Autodesk Inventor part; units mm, degrees
(part 2 of 3)
  line L626 (-3.7114, -1.0079) -> (-3.7114, -1.9201)
  line L627 (-3.7114, -1.9201) -> (-3.9151, -1.9201)
  line L628 (15.624, -5.9598) -> (15.8032, -5.9598)
  line L629 (15.8032, -5.9598) -> (15.0783, -8.4358)
  line L630 (15.0783, -8.4358) -> (14.8991, -8.4358)
  line L631 (14.8991, -8.4358) -> (15.624, -5.9598)
  line L632 (16.8294, -9.4213) -> (17.0005, -9.4213)
  line L633 (17.0005, -9.4213) -> (16.2837, -11.8973)
  line L634 (16.2837, -11.8973) -> (16.1045, -11.8973)
  line L635 (16.1045, -11.8973) -> (16.8294, -9.4213)
  line L636 (16.7006, -8.1166) -> (16.3044, -8.3052) construction
  spline S44 degree 4 poles (16.6258, -6.9128) (16.5928, -6.7161) (16.4312, -6.6396) (16.2892, -6.6526) (16.1527, -6.7477) (16.117, -6.9928) (16.263, -7.1451) (16.5325, -7.2135) (16.7006, -7.2932) (16.8664, -7.4592) (16.9149, -7.8453) (16.7006, -8.1166) (16.3044, -8.3052) (15.9635, -8.063) (15.8692, -7.8103) (15.8602, -7.6295) knots 1 1 1 1 1 2 3 4 5 6 7 8 9 10 11 12 13 13 13 13 13
  line L637 (16.6258, -6.9128) -> (16.5928, -6.7161) construction
  line L638 (16.5928, -6.7161) -> (16.4312, -6.6396) construction
  line L639 (16.4312, -6.6396) -> (16.2892, -6.6526) construction
  line L640 (16.2892, -6.6526) -> (16.1527, -6.7477) construction
  line L641 (16.1527, -6.7477) -> (16.117, -6.9928) construction
  line L642 (16.117, -6.9928) -> (16.263, -7.1451) construction
  line L643 (16.263, -7.1451) -> (16.5325, -7.2135) construction
  line L644 (16.5325, -7.2135) -> (16.7006, -7.2932) construction
  line L645 (16.7006, -7.2932) -> (16.8664, -7.4592) construction
  line L646 (16.8664, -7.4592) -> (16.9149, -7.8453) construction
  line L647 (16.9149, -7.8453) -> (16.7006, -8.1166) construction
  line L648 (16.3044, -8.3052) -> (15.9635, -8.063) construction
  line L649 (15.9635, -8.063) -> (15.8692, -7.8103) construction
  line L650 (15.8692, -7.8103) -> (15.8602, -7.6295) construction
  line L651 (16.3801, -7.4011) -> (16.1104, -7.3258) construction
  spline S45 degree 4 poles (16.072, -7.6295) (16.0903, -7.8128) (16.1895, -7.9615) (16.3888, -8.02) (16.5928, -7.9509) (16.6874, -7.7036) (16.5928, -7.5208) (16.5342, -7.4592) (16.3801, -7.4011) (16.1104, -7.3258) (15.924, -7.1016) (15.9359, -6.9137) (15.9559, -6.7161) (16.0588, -6.563) (16.226, -6.4563) (16.5549, -6.4563) (16.6874, -6.5163) (16.8173, -6.6705) (16.8457, -6.9128) knots 1 1 1 1 1 2 3 4 5 6 7 8 9 10 11 12 13 14 15 16 16 16 16 16
  line L652 (16.072, -7.6295) -> (16.0903, -7.8128) construction
  line L653 (16.0903, -7.8128) -> (16.1895, -7.9615) construction
  line L654 (16.1895, -7.9615) -> (16.3888, -8.02) construction
  line L655 (16.3888, -8.02) -> (16.5928, -7.9509) construction
  line L656 (16.5928, -7.9509) -> (16.6874, -7.7036) construction
  line L657 (16.6874, -7.7036) -> (16.5928, -7.5208) construction
  line L658 (16.5928, -7.5208) -> (16.5342, -7.4592) construction
  line L659 (16.5342, -7.4592) -> (16.3801, -7.4011) construction
  line L660 (16.1104, -7.3258) -> (15.924, -7.1016) construction
  line L661 (15.924, -7.1016) -> (15.9359, -6.9137) construction
  line L662 (15.9359, -6.9137) -> (15.9559, -6.7161) construction
  line L663 (15.9559, -6.7161) -> (16.0588, -6.563) construction
  line L664 (16.0588, -6.563) -> (16.226, -6.4563) construction
  line L665 (16.226, -6.4563) -> (16.5549, -6.4563) construction
  line L666 (16.5549, -6.4563) -> (16.6874, -6.5163) construction
  line L667 (16.6874, -6.5163) -> (16.8173, -6.6705) construction
  line L668 (16.8173, -6.6705) -> (16.8457, -6.9128) construction
  line L669 (16.6258, -6.9128) -> (16.8457, -6.9128)
  line L670 (15.8602, -7.6295) -> (16.072, -7.6295)
  line L671 (12.3499, -9.4213) -> (12.3499, -11.6122)
  line L672 (12.3499, -11.6122) -> (12.5535, -11.6122)
  line L673 (12.5535, -11.6122) -> (12.5535, -10.7624)
  line L674 (13.2295, -11.6122) -> (13.4901, -11.6122)
  line L675 (13.4901, -11.6122) -> (12.7815, -10.7245)
  line L676 (12.7815, -10.7245) -> (13.3598, -9.9507)
  line L677 (13.3598, -9.9507) -> (13.1317, -9.9507)
  line L678 (12.5535, -10.7124) -> (12.5535, -9.4213)
  line L679 (12.5535, -9.4213) -> (12.3499, -9.4213)
  line L680 (12.5535, -10.7124) -> (12.5625, -10.7124)
  line L681 (12.5625, -10.7124) -> (13.1317, -9.9507)
  line L682 (12.5535, -10.7624) -> (12.564, -10.7624)
  line L683 (12.564, -10.7624) -> (13.2295, -11.6122)
  line L684 (19.6312, -4.8847) -> (20.7633, -2.6042)
  line L685 (20.7633, -2.6042) -> (20.5923, -2.6042)
  line L686 (20.5923, -2.6042) -> (19.4602, -4.8847)
  line L687 (19.4602, -4.8847) -> (19.6312, -4.8847)
  circle A1 centre (19.4602, -3.1424) radius 0.3325
  circle A2 centre (19.4602, -3.1424) radius 0.5381
  circle A3 centre (20.7583, -4.3418) radius 0.3325
  circle A4 centre (20.7583, -4.3418) radius 0.5381
  line L688 (10.8197, 1.0564) -> (-20.3114, 1.0564)
  line L689 (-20.3114, 1.0564) -> (-20.3114, 1.2564)
  line L690 (-20.3114, 1.2564) -> (10.8197, 1.2564)
  line L691 (10.8197, 1.2564) -> (10.8197, 1.0564)
  line L692 (-21.284, 2.029) -> (-21.084, 2.029)
  line L693 (-21.084, 2.029) -> (-21.084, 12.0899)
  line L694 (-21.084, 12.0899) -> (-21.284, 12.0899)
  line L695 (-21.284, 12.0899) -> (-21.284, 2.029)
  line L696 (-20.3114, 12.8625) -> (10.8197, 12.8625)
  line L697 (10.8197, 12.8625) -> (10.8197, 13.0625)
  line L698 (10.8197, 13.0625) -> (-20.3114, 13.0625)
  line L699 (-20.3114, 13.0625) -> (-20.3114, 12.8625)
  line L700 (11.5924, 12.0899) -> (11.7924, 12.0899)
  line L701 (11.7924, 12.0899) -> (11.7924, 2.029)
  line L702 (11.7924, 2.029) -> (11.5924, 2.029)
  line L703 (11.5924, 2.029) -> (11.5924, 12.0899)
  line L704 (9.8564, 15.8189) -> (9.8564, 13.8208)
  line L705 (9.9764, 15.8189) -> (9.9764, 13.8208)
  line L706 (10.1798, 16.1424) -> (10.5173, 16.1424)
  line L707 (10.1798, 16.0224) -> (11.4983, 16.0224)
  line L708 (11.1689, 16.1424) -> (11.4983, 16.1424)
  line L709 (11.1689, 16.1424) -> (11.1689, 16.3297)
  line L710 (10.5173, 16.1424) -> (10.5173, 16.3297)
  line L711 (10.5417, 16.3541) -> (11.1444, 16.3541)
  arc A5 (10.1798, 16.1424) -> (9.8564, 15.8189) centre (10.1798, 15.8189) ccw
  arc A6 (10.1798, 16.0224) -> (9.9764, 15.8189) centre (10.1798, 15.8189) ccw
  arc A7 (11.8217, 15.8189) -> (11.4983, 16.1424) centre (11.4983, 15.8189) ccw
  arc A8 (11.7017, 15.8189) -> (11.4983, 16.0224) centre (11.4983, 15.8189) ccw
  arc A9 (9.8564, 13.8208) -> (10.1798, 13.4974) centre (10.1798, 13.8208) ccw
  arc A10 (9.9764, 13.8208) -> (10.1798, 13.6174) centre (10.1798, 13.8208) ccw
  arc A11 (11.4983, 13.6174) -> (11.7017, 13.8208) centre (11.4983, 13.8208) ccw
  arc A12 (11.4983, 13.4974) -> (11.8217, 13.8208) centre (11.4983, 13.8208) ccw
  line L712 (11.7017, 15.8189) -> (11.7017, 13.8208)
  line L713 (11.8217, 15.8189) -> (11.8217, 13.8208)
  line L714 (11.4983, 13.6174) -> (11.039, 13.6174)
  line L715 (11.039, 13.6174) -> (11.039, 13.4974)
  line L716 (11.039, 13.4974) -> (11.4983, 13.4974)
  line L717 (10.1798, 13.6174) -> (10.639, 13.6174)
  line L718 (10.639, 13.6174) -> (10.639, 13.4974)
  line L719 (10.639, 13.4974) -> (10.1798, 13.4974)
  arc A13 (10.5417, 16.3541) -> (10.5173, 16.3297) centre (10.5417, 16.3297) ccw
  arc A14 (11.1689, 16.3297) -> (11.1444, 16.3541) centre (11.1444, 16.3297) ccw
  circle A15 centre (8.2981, 11.6945) radius 0.3325
  circle A16 centre (8.2981, 11.6945) radius 0.5381
  line L720 (9.597, 7.7802) -> (8.7499, 5.345)
  line L721 (8.7499, 5.345) -> (10.4521, 5.345)
  line L722 (10.4521, 5.345) -> (9.597, 7.7802)
  line L723 (8.7499, 4.4979) -> (10.4521, 4.4979)
  line L724 (10.4521, 4.4979) -> (9.597, 2.0627)
  line L725 (9.597, 2.0627) -> (8.7499, 4.4979)
  line L726 (9.3608, 5.295) -> (9.8413, 5.295)
  line L727 (9.8413, 5.295) -> (9.8413, 4.5479)
  line L728 (9.8413, 4.5479) -> (9.3608, 4.5479)
  line L729 (9.3608, 4.5479) -> (9.3608, 5.295)
  line L730 (13.8648, -0.8287) -> (16.3, 0.0184)
  line L731 (16.3, 0.0184) -> (16.3, -1.6839)
  line L732 (16.3, -1.6839) -> (13.8648, -0.8287)
  line L733 (17.8068, 0.0591) -> (20.242, -0.788)
  line L734 (20.242, -0.788) -> (17.8068, -1.6432)
  line L735 (17.8068, -1.6432) -> (17.8068, 0.0591)
  line L736 (16.35, -0.5925) -> (17.7568, -0.5925)
  line L737 (17.7568, -0.5925) -> (17.7568, -1.073)
  line L738 (17.7568, -1.073) -> (16.35, -1.073)
  line L739 (16.35, -1.073) -> (16.35, -0.5925)
  line L740 (-21.0759, -3.4746) -> (-20.8759, -3.4746)
  line L741 (-20.8759, -3.4746) -> (-20.8759, -10.636)
  line L742 (-20.8759, -10.636) -> (-21.0759, -10.636)
  line L743 (-21.0759, -10.636) -> (-21.0759, -3.4746)
  line L744 (-20.1032, -11.2086) -> (-0.5783, -11.2086)
  line L745 (-0.5783, -11.2086) -> (-0.5783, -11.4086)
  line L746 (-0.5783, -11.4086) -> (-20.1032, -11.4086)
  line L747 (-20.1032, -11.4086) -> (-20.1032, -11.2086)
  line L748 (1.167, -11.2086) -> (10.6197, -11.2086)
  line L749 (10.6197, -11.2086) -> (10.6197, -11.4086)
  line L750 (10.6197, -11.4086) -> (1.167, -11.4086)
  line L751 (1.167, -11.4086) -> (1.167, -11.2086)
  line L752 (11.3924, -3.4746) -> (11.5924, -3.4746)
  line L753 (11.5924, -3.4746) -> (11.5924, -10.636)
  line L754 (11.5924, -10.636) -> (11.3924, -10.636)
  line L755 (11.3924, -10.636) -> (11.3924, -3.4746)
  line L756 (1.167, -2.702) -> (10.6197, -2.702)
  line L757 (10.6197, -2.702) -> (10.6197, -2.902)
  line L758 (10.6197, -2.902) -> (1.167, -2.902)
  line L759 (1.167, -2.902) -> (1.167, -2.702)
  line L760 (0.1943, -3.4746) -> (0.3943, -3.4746)
  line L761 (0.3943, -3.4746) -> (0.3943, -10.636)
  line L762 (0.3943, -10.636) -> (0.1943, -10.636)
  line L763 (0.1943, -10.636) -> (0.1943, -3.4746)
  line L764 (-20.1032, -2.702) -> (-0.5783, -2.702)
  line L765 (-0.5783, -2.702) -> (-0.5783, -2.902)
  line L766 (-0.5783, -2.902) -> (-20.1032, -2.902)
  line L767 (-20.1032, -2.902) -> (-20.1032, -2.702)
  line L768 (5.5409, -9.6819) -> (6.2658, -9.6819)
  line L769 (6.2658, -9.6819) -> (6.2658, -10.3987)
  line L770 (6.2658, -10.3987) -> (5.5409, -10.3987)
  line L771 (5.5409, -10.3987) -> (5.5409, -9.6819)
  line L772 (-10.9195, -5.7806) -> (-10.1946, -5.7806)
  line L773 (-10.1946, -5.7806) -> (-10.1946, -6.5055)
  line L774 (-10.1946, -6.5055) -> (-10.9195, -6.5055)
  line L775 (-10.9195, -6.5055) -> (-10.9195, -5.7806)
  line L776 (-10.9195, -7.5236) -> (-10.1946, -7.5236)
  line L777 (-10.1946, -7.5236) -> (-10.1946, -8.2403)
  line L778 (-10.1946, -8.2403) -> (-10.9195, -8.2403)
  line L779 (-10.9195, -8.2403) -> (-10.9195, -7.5236)
  line L780 (-10.9195, -9.6819) -> (-10.1946, -9.6819)
  line L781 (-10.1946, -9.6819) -> (-10.1946, -10.3987)
  line L782 (-10.1946, -10.3987) -> (-10.9195, -10.3987)
  line L783 (-10.9195, -10.3987) -> (-10.9195, -9.6819)
  line L784 (-5.7558, -9.6819) -> (-5.0309, -9.6819)
  line L785 (-5.0309, -9.6819) -> (-5.0309, -10.3987)
  line L786 (-5.0309, -10.3987) -> (-5.7558, -10.3987)
  line L787 (-5.7558, -10.3987) -> (-5.7558, -9.6819)
  line L788 (-19.4714, -3.6467) -> (-17.2723, -3.6467)
  line L789 (-17.2723, -3.6467) -> (-16.9221, -3.997)
  line L790 (-16.9221, -3.997) -> (-17.2397, -4.3146)
  line L791 (-17.2397, -4.3146) -> (-19.4567, -4.3146)
  line L792 (-19.7938, -3.9691) -> (-19.4714, -3.6467)
  line L793 (-19.8786, -4.054) -> (-19.5528, -4.3879)
  line L794 (-19.5528, -4.3879) -> (-19.5528, -6.5964)
  line L795 (-19.5528, -6.5964) -> (-19.9227, -6.9664)
  line L796 (-19.9227, -6.9664) -> (-20.2125, -6.6766)
  line L797 (-20.2125, -6.6766) -> (-20.2125, -4.3879)
  line L798 (-20.2125, -4.3879) -> (-19.8786, -4.054)
  line L799 (-19.8379, -7.0512) -> (-19.504, -6.7173)
  line L800 (-19.504, -6.7173) -> (-17.2397, -6.7173)
  line L801 (-17.2397, -6.7173) -> (-16.9058, -7.0512)
  line L802 (-16.9058, -7.0512) -> (-17.2397, -7.3851)
  line L803 (-17.2397, -7.3851) -> (-19.504, -7.3851)
  line L804 (-19.504, -7.3851) -> (-19.8379, -7.0512)
  line L805 (-19.7938, -3.9691) -> (-19.4567, -4.3146)
  line L806 (-16.8372, -4.0818) -> (-17.199, -4.4436)
  line L807 (-17.199, -4.4436) -> (-17.199, -6.5883)
  line L808 (-17.199, -6.5883) -> (-16.821, -6.9664)
  line L809 (-16.821, -6.9664) -> (-16.5312, -6.6766)
  line L810 (-16.5312, -6.6766) -> (-16.5312, -4.3879)
  line L811 (-16.5312, -4.3879) -> (-16.8372, -4.0818)
  line L812 (-16.821, -7.1361) -> (-17.199, -7.5141)
  line L813 (-17.199, -7.5141) -> (-17.199, -9.7064)
  line L814 (-17.199, -9.7064) -> (-16.8651, -10.0403)
  line L815 (-16.8651, -10.0403) -> (-16.5312, -9.7064)
  line L816 (-16.5312, -9.7064) -> (-16.5312, -7.4259)
  line L817 (-16.5312, -7.4259) -> (-16.821, -7.1361)
  line L818 (-19.9227, -7.1361) -> (-20.2125, -7.4259)
  line L819 (-20.2125, -7.4259) -> (-20.2125, -9.7064)
  line L820 (-20.2125, -9.7064) -> (-19.8786, -10.0403)
  line L821 (-19.8786, -10.0403) -> (-19.5528, -9.7064)
  line L822 (-19.5528, -9.7064) -> (-19.5528, -7.506)
  line L823 (-19.5528, -7.506) -> (-19.9227, -7.1361)
  line L824 (-19.7938, -10.1252) -> (-19.417, -9.739)
  line L825 (-19.417, -9.739) -> (-17.3361, -9.739)
  line L826 (-17.3361, -9.739) -> (-16.9499, -10.1252)
  line L827 (-16.9499, -10.1252) -> (-17.2316, -10.4068)
  line L828 (-17.2316, -10.4068) -> (-19.5121, -10.4068)
  line L829 (-19.5121, -10.4068) -> (-19.7938, -10.1252)
  line L830 (-11.6919, -4.0818) -> (-12.0536, -4.4436)
  line L831 (-11.6756, -7.1361) -> (-12.0536, -7.5141)
  line L832 (-11.7604, -7.0512) -> (-12.0943, -7.3851)
  line L833 (-14.4074, -9.7064) -> (-14.4074, -7.506)
  line L834 (-15.0672, -7.4259) -> (-15.0672, -9.7064)
  line L835 (-14.7774, -7.1361) -> (-15.0672, -7.4259)
  line L836 (-14.4074, -7.506) -> (-14.7774, -7.1361)
  line L837 (-14.3586, -7.3851) -> (-14.6925, -7.0512)
  line L838 (-12.0943, -7.3851) -> (-14.3586, -7.3851)
  line L839 (-11.3858, -6.6766) -> (-11.3858, -4.3879)
  line L840 (-11.6756, -6.9664) -> (-11.3858, -6.6766)
  line L841 (-11.3858, -7.4259) -> (-11.6756, -7.1361)
  line L842 (-11.3858, -9.7064) -> (-11.3858, -7.4259)
  line L843 (-12.0536, -7.5141) -> (-12.0536, -9.7064)
  line L844 (-11.3858, -4.3879) -> (-11.6919, -4.0818)
  line L845 (-14.6484, -3.9691) -> (-14.326, -3.6467)
  line L846 (-14.6484, -3.9691) -> (-14.3113, -4.3146)
  line L847 (-14.7332, -4.054) -> (-14.4074, -4.3879)
  line L848 (-15.0672, -4.3879) -> (-14.7332, -4.054)
  line L849 (-14.326, -3.6467) -> (-12.1269, -3.6467)
  line L850 (-12.1269, -3.6467) -> (-11.7767, -3.997)
  line L851 (-12.0943, -4.3146) -> (-14.3113, -4.3146)
  line L852 (-11.7767, -3.997) -> (-12.0943, -4.3146)
  line L853 (-12.0536, -4.4436) -> (-12.0536, -6.5883)
  line L854 (-14.3586, -6.7173) -> (-12.0943, -6.7173)
  line L855 (-12.0536, -6.5883) -> (-11.6756, -6.9664)
  line L856 (-12.0943, -6.7173) -> (-11.7604, -7.0512)
  line L857 (-14.4074, -4.3879) -> (-14.4074, -6.5964)
  line L858 (-15.0672, -6.6766) -> (-15.0672, -4.3879)
  line L859 (-14.6925, -7.0512) -> (-14.3586, -6.7173)
  line L860 (-14.4074, -6.5964) -> (-14.7774, -6.9664)
  line L861 (-14.7774, -6.9664) -> (-15.0672, -6.6766)
  line L862 (-14.2716, -9.739) -> (-12.1908, -9.739)
  line L863 (-11.7197, -10.0403) -> (-11.3858, -9.7064)
  line L864 (-12.0536, -9.7064) -> (-11.7197, -10.0403)
  line L865 (-12.1908, -9.739) -> (-11.8045, -10.1252)
  line L866 (-12.0862, -10.4068) -> (-14.3667, -10.4068)
  line L867 (-11.8045, -10.1252) -> (-12.0862, -10.4068)
  line L868 (-14.7332, -10.0403) -> (-14.4074, -9.7064)
  line L869 (-14.6484, -10.1252) -> (-14.2716, -9.739)
  line L870 (-15.0672, -9.7064) -> (-14.7332, -10.0403)
  line L871 (-14.3667, -10.4068) -> (-14.6484, -10.1252)
  line L872 (-6.4446, -4.0818) -> (-6.8064, -4.4436)
  line L873 (-6.4284, -7.1361) -> (-6.8064, -7.5141)
  line L874 (-6.5132, -7.0512) -> (-6.8471, -7.3851)
  line L875 (-9.1602, -9.7064) -> (-9.1602, -7.506)
  line L876 (-9.8199, -7.4259) -> (-9.8199, -9.7064)
  line L877 (-9.5301, -7.1361) -> (-9.8199, -7.4259)
  line L878 (-9.1602, -7.506) -> (-9.5301, -7.1361)
  line L879 (-9.1114, -7.3851) -> (-9.4453, -7.0512)
  line L880 (-6.8471, -7.3851) -> (-9.1114, -7.3851)
  line L881 (-6.1386, -6.6766) -> (-6.1386, -4.3879)
  line L882 (-6.4284, -6.9664) -> (-6.1386, -6.6766)
  line L883 (-6.1386, -7.4259) -> (-6.4284, -7.1361)
  line L884 (-6.1386, -9.7064) -> (-6.1386, -7.4259)
  line L885 (-6.8064, -7.5141) -> (-6.8064, -9.7064)
  line L886 (-6.1386, -4.3879) -> (-6.4446, -4.0818)
  line L887 (-9.4012, -3.9691) -> (-9.0788, -3.6467)
  line L888 (-9.4012, -3.9691) -> (-9.0641, -4.3146)
  line L889 (-9.486, -4.054) -> (-9.1602, -4.3879)
  line L890 (-9.8199, -4.3879) -> (-9.486, -4.054)
  line L891 (-9.0788, -3.6467) -> (-6.8797, -3.6467)
  line L892 (-6.8797, -3.6467) -> (-6.5295, -3.997)
  line L893 (-6.8471, -4.3146) -> (-9.0641, -4.3146)
  line L894 (-6.5295, -3.997) -> (-6.8471, -4.3146)
  line L895 (-6.8064, -4.4436) -> (-6.8064, -6.5883)
  line L896 (-9.1114, -6.7173) -> (-6.8471, -6.7173)
  line L897 (-6.8064, -6.5883) -> (-6.4284, -6.9664)
  line L898 (-6.8471, -6.7173) -> (-6.5132, -7.0512)
  line L899 (-9.1602, -4.3879) -> (-9.1602, -6.5964)
  line L900 (-9.8199, -6.6766) -> (-9.8199, -4.3879)
  line L901 (-9.4453, -7.0512) -> (-9.1114, -6.7173)
  line L902 (-9.1602, -6.5964) -> (-9.5301, -6.9664)
  line L903 (-9.5301, -6.9664) -> (-9.8199, -6.6766)
  line L904 (-9.0244, -9.739) -> (-6.9435, -9.739)
  line L905 (-6.4725, -10.0403) -> (-6.1386, -9.7064)
  line L906 (-6.8064, -9.7064) -> (-6.4725, -10.0403)
  line L907 (-6.9435, -9.739) -> (-6.5573, -10.1252)
  line L908 (-6.839, -10.4068) -> (-9.1195, -10.4068)
  line L909 (-6.5573, -10.1252) -> (-6.839, -10.4068)
  line L910 (-9.486, -10.0403) -> (-9.1602, -9.7064)
  line L911 (-9.4012, -10.1252) -> (-9.0244, -9.739)
  line L912 (-9.8199, -9.7064) -> (-9.486, -10.0403)
  line L913 (-9.1195, -10.4068) -> (-9.4012, -10.1252)
  line L914 (-1.2565, -4.0818) -> (-1.6183, -4.4436)
  line L915 (-1.2402, -7.1361) -> (-1.6183, -7.5141)
  line L916 (-1.325, -7.0512) -> (-1.659, -7.3851)
  line L917 (-3.9721, -9.7064) -> (-3.9721, -7.506)
  line L918 (-4.6318, -7.4259) -> (-4.6318, -9.7064)
  line L919 (-4.342, -7.1361) -> (-4.6318, -7.4259)
  line L920 (-3.9721, -7.506) -> (-4.342, -7.1361)
  line L921 (-3.9232, -7.3851) -> (-4.2571, -7.0512)
  line L922 (-1.659, -7.3851) -> (-3.9232, -7.3851)
  line L923 (-0.9504, -6.6766) -> (-0.9504, -4.3879)
  line L924 (-1.2402, -6.9664) -> (-0.9504, -6.6766)
  line L925 (-0.9504, -7.4259) -> (-1.2402, -7.1361)
  line L926 (-0.9504, -9.7064) -> (-0.9504, -7.4259)
  line L927 (-1.6183, -7.5141) -> (-1.6183, -9.7064)
  line L928 (-0.9504, -4.3879) -> (-1.2565, -4.0818)
  line L929 (-4.213, -3.9691) -> (-3.8906, -3.6467)
  line L930 (-4.213, -3.9691) -> (-3.8759, -4.3146)
  line L931 (-4.2979, -4.054) -> (-3.9721, -4.3879)
  line L932 (-4.6318, -4.3879) -> (-4.2979, -4.054)
  line L933 (-3.8906, -3.6467) -> (-1.6916, -3.6467)
  line L934 (-1.6916, -3.6467) -> (-1.3413, -3.997)
  line L935 (-1.659, -4.3146) -> (-3.8759, -4.3146)
  line L936 (-1.3413, -3.997) -> (-1.659, -4.3146)
  line L937 (-1.6183, -4.4436) -> (-1.6183, -6.5883)
  line L938 (-3.9232, -6.7173) -> (-1.659, -6.7173)
  line L939 (-1.6183, -6.5883) -> (-1.2402, -6.9664)
  line L940 (-1.659, -6.7173) -> (-1.325, -7.0512)
  line L941 (-3.9721, -4.3879) -> (-3.9721, -6.5964)
  line L942 (-4.6318, -6.6766) -> (-4.6318, -4.3879)
  line L943 (-4.2571, -7.0512) -> (-3.9232, -6.7173)
  line L944 (-3.9721, -6.5964) -> (-4.342, -6.9664)
  line L945 (-4.342, -6.9664) -> (-4.6318, -6.6766)
  line L946 (-3.8362, -9.739) -> (-1.7554, -9.739)
  line L947 (-1.2843, -10.0403) -> (-0.9504, -9.7064)
  line L948 (-1.6183, -9.7064) -> (-1.2843, -10.0403)
  line L949 (-1.7554, -9.739) -> (-1.3692, -10.1252)
  line L950 (-1.6508, -10.4068) -> (-3.9313, -10.4068)
  line L951 (-1.3692, -10.1252) -> (-1.6508, -10.4068)
  line L952 (-4.2979, -10.0403) -> (-3.9721, -9.7064)
  line L953 (-4.213, -10.1252) -> (-3.8362, -9.739)
  line L954 (-4.6318, -9.7064) -> (-4.2979, -10.0403)
  line L955 (-3.9313, -10.4068) -> (-4.213, -10.1252)
  line L956 (4.8439, -4.0818) -> (4.4821, -4.4436)
  line L957 (4.8602, -7.1361) -> (4.4821, -7.5141)
  line L958 (4.7753, -7.0512) -> (4.4414, -7.3851)
  line L959 (2.1283, -9.7064) -> (2.1283, -7.506)
  line L960 (1.4686, -7.4259) -> (1.4686, -9.7064)
  line L961 (1.7584, -7.1361) -> (1.4686, -7.4259)
  line L962 (2.1283, -7.506) -> (1.7584, -7.1361)
  line L963 (2.1772, -7.3851) -> (1.8432, -7.0512)
  line L964 (4.4414, -7.3851) -> (2.1772, -7.3851)
  line L965 (5.15, -6.6766) -> (5.15, -4.3879)
  line L966 (4.8602, -6.9664) -> (5.15, -6.6766)
  line L967 (5.15, -7.4259) -> (4.8602, -7.1361)
  line L968 (5.15, -9.7064) -> (5.15, -7.4259)
  line L969 (4.4821, -7.5141) -> (4.4821, -9.7064)
  line L970 (5.15, -4.3879) -> (4.8439, -4.0818)
  line L971 (1.8874, -3.9691) -> (2.2097, -3.6467)
  line L972 (1.8874, -3.9691) -> (2.2244, -4.3146)
  line L973 (1.8025, -4.054) -> (2.1283, -4.3879)
  line L974 (1.4686, -4.3879) -> (1.8025, -4.054)
  line L975 (2.2097, -3.6467) -> (4.4088, -3.6467)
  line L976 (4.4088, -3.6467) -> (4.759, -3.997)
  line L977 (4.4414, -4.3146) -> (2.2244, -4.3146)
  line L978 (4.759, -3.997) -> (4.4414, -4.3146)
  line L979 (4.4821, -4.4436) -> (4.4821, -6.5883)
  line L980 (2.1772, -6.7173) -> (4.4414, -6.7173)
  line L981 (4.4821, -6.5883) -> (4.8602, -6.9664)
  line L982 (4.4414, -6.7173) -> (4.7753, -7.0512)
  line L983 (2.1283, -4.3879) -> (2.1283, -6.5964)
  line L984 (1.4686, -6.6766) -> (1.4686, -4.3879)
  line L985 (1.8432, -7.0512) -> (2.1772, -6.7173)
  line L986 (2.1283, -6.5964) -> (1.7584, -6.9664)
  line L987 (1.7584, -6.9664) -> (1.4686, -6.6766)
  line L988 (2.2642, -9.739) -> (4.345, -9.739)
  line L989 (4.816, -10.0403) -> (5.15, -9.7064)
  line L990 (4.4821, -9.7064) -> (4.816, -10.0403)
  line L991 (4.345, -9.739) -> (4.7312, -10.1252)
  line L992 (4.4495, -10.4068) -> (2.169, -10.4068)
  line L993 (4.7312, -10.1252) -> (4.4495, -10.4068)
  line L994 (1.8025, -10.0403) -> (2.1283, -9.7064)
  line L995 (1.8874, -10.1252) -> (2.2642, -9.739)
  line L996 (1.4686, -9.7064) -> (1.8025, -10.0403)
  line L997 (2.169, -10.4068) -> (1.8874, -10.1252)
  line L998 (10.032, -4.0818) -> (9.6703, -4.4436)
  line L999 (10.0483, -7.1361) -> (9.6703, -7.5141)
  line L1000 (9.9635, -7.0512) -> (9.6295, -7.3851)
  line L1001 (7.3164, -9.7064) -> (7.3164, -7.506)
  line L1002 (6.6567, -7.4259) -> (6.6567, -9.7064)
  line L1003 (6.9465, -7.1361) -> (6.6567, -7.4259)
  line L1004 (7.3164, -7.506) -> (6.9465, -7.1361)
  line L1005 (7.3653, -7.3851) -> (7.0314, -7.0512)
  line L1006 (9.6295, -7.3851) -> (7.3653, -7.3851)
  line L1007 (10.3381, -6.6766) -> (10.3381, -4.3879)
  line L1008 (10.0483, -6.9664) -> (10.3381, -6.6766)
  line L1009 (10.3381, -7.4259) -> (10.0483, -7.1361)
  line L1010 (10.3381, -9.7064) -> (10.3381, -7.4259)
  line L1011 (9.6703, -7.5141) -> (9.6703, -9.7064)
  line L1012 (10.3381, -4.3879) -> (10.032, -4.0818)
  line L1013 (7.0755, -3.9691) -> (7.3979, -3.6467)
  line L1014 (7.0755, -3.9691) -> (7.4126, -4.3146)
  line L1015 (6.9907, -4.054) -> (7.3164, -4.3879)
  line L1016 (6.6567, -4.3879) -> (6.9907, -4.054)
  line L1017 (7.3979, -3.6467) -> (9.597, -3.6467)
  line L1018 (9.597, -3.6467) -> (9.9472, -3.997)
  line L1019 (9.6295, -4.3146) -> (7.4126, -4.3146)
  line L1020 (9.9472, -3.997) -> (9.6295, -4.3146)
  line L1021 (9.6703, -4.4436) -> (9.6703, -6.5883)
  line L1022 (7.3653, -6.7173) -> (9.6295, -6.7173)
  line L1023 (9.6703, -6.5883) -> (10.0483, -6.9664)
  line L1024 (9.6295, -6.7173) -> (9.9635, -7.0512)
  line L1025 (7.3164, -4.3879) -> (7.3164, -6.5964)
  line L1026 (6.6567, -6.6766) -> (6.6567, -4.3879)
  line L1027 (7.0314, -7.0512) -> (7.3653, -6.7173)
  line L1028 (7.3164, -6.5964) -> (6.9465, -6.9664)
  line L1029 (6.9465, -6.9664) -> (6.6567, -6.6766)
  line L1030 (7.4523, -9.739) -> (9.5331, -9.739)
  line L1031 (10.0042, -10.0403) -> (10.3381, -9.7064)
  line L1032 (9.6703, -9.7064) -> (10.0042, -10.0403)
  line L1033 (9.5331, -9.739) -> (9.9193, -10.1252)
  line L1034 (9.6377, -10.4068) -> (7.3572, -10.4068)
  line L1035 (9.9193, -10.1252) -> (9.6377, -10.4068)
  line L1036 (6.9907, -10.0403) -> (7.3164, -9.7064)
  line L1037 (7.0755, -10.1252) -> (7.4523, -9.739)
  line L1038 (6.6567, -9.7064) -> (6.9907, -10.0403)
  line L1039 (7.3572, -10.4068) -> (7.0755, -10.1252)
  line L1040 (8.8351, 11.1064) -> (8.8351, 8.9128)
  line L1041 (9.3135, 11.0282) -> (9.3135, 8.9574)
  line L1042 (9.3986, 11.5912) -> (10.3586, 11.5912)
  line L1043 (9.4283, 11.1129) -> (10.3586, 11.1129)
  line L1044 (8.8351, 11.1064) -> (8.9706, 11.5358) construction
  line L1045 (8.9706, 11.5358) -> (9.3986, 11.5912) construction
  spline S46 degree 2 poles (8.8351, 11.1064) (8.9706, 11.5358) (9.3986, 11.5912) knots 1 1 1 2 2 2
  line L1046 (9.3135, 11.0282) -> (9.3594, 11.1062) construction
  line L1047 (9.3594, 11.1062) -> (9.4283, 11.1129) construction
  spline S47 degree 2 poles (9.3135, 11.0282) (9.3594, 11.1062) (9.4283, 11.1129) knots 1 1 1 2 2 2
  line L1048 (8.8351, 8.9128) -> (8.9277, 8.4536) construction
  line L1049 (8.9277, 8.4536) -> (9.3729, 8.3522) construction
  spline S48 degree 2 poles (8.8351, 8.9128) (8.9277, 8.4536) (9.3729, 8.3522) knots 1 1 1 2 2 2
  line L1050 (9.3135, 8.9574) -> (9.3317, 8.865) construction
  line L1051 (9.3317, 8.865) -> (9.4306, 8.8306) construction
  spline S49 degree 2 poles (9.3135, 8.9574) (9.3317, 8.865) (9.4306, 8.8306) knots 1 1 1 2 2 2
  line L1052 (10.386, 8.8306) -> (10.5862, 8.7305) construction
  line L1053 (10.5862, 8.7305) -> (10.5862, 8.4536) construction
  line L1054 (10.5862, 8.4536) -> (10.386, 8.3522) construction
  spline S50 degree 3 poles (10.386, 8.8306) (10.5862, 8.7305) (10.5862, 8.4536) (10.386, 8.3522) knots 1 1 1 1 2 2 2 2
  line L1055 (10.3586, 11.5912) -> (10.611, 11.5234) construction
  line L1056 (10.611, 11.5234) -> (10.611, 11.1907) construction
  line L1057 (10.611, 11.1907) -> (10.3586, 11.1129) construction
  spline S51 degree 3 poles (10.3586, 11.5912) (10.611, 11.5234) (10.611, 11.1907) (10.3586, 11.1129) knots 1 1 1 1 2 2 2 2
  line L1058 (9.4306, 8.8306) -> (10.386, 8.8306)
  line L1059 (10.386, 8.3522) -> (9.3729, 8.3522)
  line L1060 (10.1264, 15.1719) -> (11.511, 15.8398)
  line L1061 (10.1264, 15.7828) -> (10.1264, 15.1719)
  line L1062 (11.4214, 15.8724) -> (10.2567, 15.8724)
  line L1063 (10.1264, 14.8158) -> (11.5517, 15.5)
  line L1064 (11.5517, 15.5) -> (11.5517, 14.824)
  line L1065 (11.5517, 14.824) -> (10.1264, 14.1398)
  line L1066 (10.1264, 14.1398) -> (10.1264, 14.8158)
  line L1067 (10.1671, 13.8) -> (11.5517, 14.4679)
  line L1068 (10.2567, 13.7674) -> (11.4214, 13.7674)
  line L1069 (10.1264, 15.7828) -> (10.1419, 15.8725) construction
  line L1070 (10.1419, 15.8725) -> (10.2567, 15.8724) construction
  spline S52 degree 2 poles (10.1264, 15.7828) (10.1419, 15.8725) (10.2567, 15.8724) knots 1 1 1 2 2 2
  line L1071 (11.4214, 15.8724) -> (11.4945, 15.8725) construction
  line L1072 (11.4945, 15.8725) -> (11.511, 15.8398) construction
  spline S53 degree 2 poles (11.4214, 15.8724) (11.4945, 15.8725) (11.511, 15.8398) knots 1 1 1 2 2 2
  line L1073 (11.5517, 14.4679) -> (11.5517, 13.8733)
  line L1074 (11.5517, 13.8733) -> (11.5412, 13.7747) construction
  line L1075 (11.5412, 13.7747) -> (11.4214, 13.7674) construction
  spline S54 degree 2 poles (11.5517, 13.8733) (11.5412, 13.7747) (11.4214, 13.7674) knots 1 1 1 2 2 2
  line L1076 (10.1671, 13.8) -> (10.2004, 13.7674) construction
  line L1077 (10.2004, 13.7674) -> (10.2567, 13.7674) construction
  spline S55 degree 2 poles (10.1671, 13.8) (10.2004, 13.7674) (10.2567, 13.7674) knots 1 1 1 2 2 2
  circle A17 centre (14.8258, 15.2163) radius 0.3393
  arc A18 (13.882, 16.4787) -> (13.482, 16.0787) centre (13.882, 16.0787) ccw
  arc A19 (16.1697, 16.0787) -> (15.7697, 16.4787) centre (15.7697, 16.0787) ccw
  arc A20 (15.7697, 13.9539) -> (16.1697, 14.3539) centre (15.7697, 14.3539) ccw
  arc A21 (13.482, 14.3539) -> (13.882, 13.9539) centre (13.882, 14.3539) ccw
  line L1078 (13.882, 16.4787) -> (15.7697, 16.4787)
  line L1079 (16.1697, 16.0787) -> (16.1697, 14.3539)
  line L1080 (15.7697, 13.9539) -> (13.882, 13.9539)
  line L1081 (13.482, 16.0787) -> (13.482, 14.3539)
  arc A22 (18.3199, 14.3132) -> (18.7199, 13.9132) centre (18.7199, 14.3132) ccw
  line L1082 (18.3199, 16.038) -> (18.3199, 14.3132)
  arc A23 (18.7199, 16.438) -> (18.3199, 16.038) centre (18.7199, 16.038) ccw
  line L1083 (20.6076, 13.9132) -> (18.7199, 13.9132)
  line L1084 (18.7199, 16.438) -> (20.6076, 16.438)
  arc A24 (20.6076, 13.9132) -> (21.0076, 14.3132) centre (20.6076, 14.3132) ccw
  line L1085 (21.0076, 16.038) -> (21.0076, 14.3132)
  arc A25 (21.0076, 16.038) -> (20.6076, 16.438) centre (20.6076, 16.038) ccw
  line L1086 (19.4351, 14.4795) -> (19.8604, 14.4795)
  line L1087 (19.8604, 14.4795) -> (19.8604, 14.113)
  line L1088 (19.8604, 14.113) -> (19.4351, 14.113)
  line L1089 (19.4351, 14.113) -> (19.4351, 14.4795)
  line L1090 (19.4125, 15.6158) -> (19.4125, 16.0107)
  line L1091 (19.4125, 16.0107) -> (19.8849, 16.0107)
  line L1092 (19.8849, 16.0107) -> (19.8849, 15.5096)
  line L1093 (19.8849, 15.5096) -> (19.7772, 14.6017)
  line L1094 (19.7772, 14.6017) -> (19.5328, 14.6017)
  line L1095 (19.5328, 14.6017) -> (19.4125, 15.6158)
  line L1096 (5.0034, 14.1331) -> (5.6549, 14.5403)
  line L1097 (5.6549, 14.5403) -> (5.6549, 13.848)
  line L1098 (5.6549, 13.848) -> (5.0034, 13.848)
  line L1099 (5.0034, 13.848) -> (5.0034, 14.1331)
  line L1100 (5.997, 14.7602) -> (6.6486, 15.1756)
  line L1101 (6.6486, 15.1756) -> (6.6486, 13.848)
  line L1102 (6.6486, 13.848) -> (5.997, 13.848)
  line L1103 (5.997, 13.848) -> (5.997, 14.7602)
  line L1104 (6.9907, 15.3874) -> (7.6422, 15.8027)
  line L1105 (7.6422, 15.8027) -> (7.6422, 13.848)
  line L1106 (7.6422, 13.848) -> (6.9907, 13.848)
  line L1107 (6.9907, 13.848) -> (6.9907, 15.3874)
  line L1108 (7.9843, 16.0226) -> (8.6359, 16.4266)
  line L1109 (8.6359, 16.4266) -> (8.6359, 13.848)
  line L1110 (8.6359, 13.848) -> (7.9843, 13.848)
  line L1111 (7.9843, 13.848) -> (7.9843, 16.0226)
  line L1112 (14.774, 4.2212) -> (14.774, 4.6384)
  line L1113 (14.774, 4.6384) -> (14.4512, 5.0436)
  line L1114 (14.4512, 5.0436) -> (14.545, 5.1184)
  line L1115 (14.545, 5.1184) -> (14.774, 4.831)
  line L1116 (14.774, 4.831) -> (14.774, 5.2309)
  line L1117 (14.774, 5.2309) -> (14.894, 5.2309)
  line L1118 (14.894, 5.2309) -> (14.894, 4.8352)
  line L1119 (14.894, 4.8352) -> (15.114, 5.1174)
  line L1120 (15.114, 5.1174) -> (15.2086, 5.0436)
  line L1121 (15.2086, 5.0436) -> (14.894, 4.64)
  line L1122 (14.894, 4.64) -> (14.894, 4.2212)
  circle A26 centre (14.834, 3.9115) radius 0.1964
  line L1123 (13.9297, 4.757) -> (14.0409, 4.802)
  line L1124 (14.2331, 4.3277) -> (14.5958, 4.1183)
  line L1125 (14.0409, 4.802) -> (14.2331, 4.3277)
  line L1126 (14.064, 4.4253) -> (13.9297, 4.757)
  line L1127 (13.7213, 4.6232) -> (14.064, 4.4253)
  line L1128 (13.6613, 4.5193) -> (13.7213, 4.6232)
  line L1129 (14.0077, 4.3193) -> (13.6613, 4.5193)
  line L1130 (13.6443, 4.2647) -> (14.0077, 4.3193)
  line L1131 (14.5358, 4.0144) -> (14.1745, 4.223)
  line L1132 (14.1745, 4.223) -> (13.6621, 4.1461)
  line L1133 (13.6621, 4.1461) -> (13.6443, 4.2647)
  line L1134 (13.6496, 3.5511) -> (13.6662, 3.6699)
  line L1135 (14.1731, 3.5992) -> (14.5358, 3.8086)
  line L1136 (13.6662, 3.6699) -> (14.1731, 3.5992)
  line L1137 (14.004, 3.5016) -> (13.6496, 3.5511)
  line L1138 (13.6613, 3.3038) -> (14.004, 3.5016)
  line L1139 (13.7213, 3.1998) -> (13.6613, 3.3038)
  line L1140 (14.0677, 3.3998) -> (13.7213, 3.1998)
  line L1141 (13.9333, 3.0578) -> (14.0677, 3.3998)
  line L1142 (14.5958, 3.7047) -> (14.2345, 3.4961)
  line L1143 (14.2345, 3.4961) -> (14.0449, 3.0139)
  line L1144 (14.0449, 3.0139) -> (13.9333, 3.0578)
  line L1145 (14.554, 2.7056) -> (14.4593, 2.7794)
  line L1146 (14.774, 3.183) -> (14.774, 3.6018)
  line L1147 (14.4593, 2.7794) -> (14.774, 3.183)
  line L1148 (14.774, 2.9878) -> (14.554, 2.7056)
  line L1149 (14.774, 2.5921) -> (14.774, 2.9878)
  line L1150 (14.894, 2.5921) -> (14.774, 2.5921)
  line L1151 (14.894, 2.992) -> (14.894, 2.5921)
  line L1152 (15.1229, 2.7046) -> (14.894, 2.992)
  line L1153 (14.894, 3.6018) -> (14.894, 3.1846)
  line L1154 (14.894, 3.1846) -> (15.2168, 2.7794)
  line L1155 (15.2168, 2.7794) -> (15.1229, 2.7046)
  line L1156 (15.7383, 3.0661) -> (15.6271, 3.021)
  line L1157 (15.4349, 3.4953) -> (15.0722, 3.7047)
  line L1158 (15.6271, 3.021) -> (15.4349, 3.4953)
  line L1159 (15.6039, 3.3977) -> (15.7383, 3.0661)
  line L1160 (15.9466, 3.1998) -> (15.6039, 3.3977)
  line L1161 (16.0066, 3.3038) -> (15.9466, 3.1998)
  line L1162 (15.6603, 3.5037) -> (16.0066, 3.3038)
  line L1163 (16.0236, 3.5583) -> (15.6603, 3.5037)
  line L1164 (15.1322, 3.8086) -> (15.4935, 3.6)
  line L1165 (15.4935, 3.6) -> (16.0058, 3.677)
  line L1166 (16.0058, 3.677) -> (16.0236, 3.5583)
  line L1167 (16.0183, 4.272) -> (16.0017, 4.1531)
  line L1168 (15.4949, 4.2238) -> (15.1322, 4.0144)
  line L1169 (16.0017, 4.1531) -> (15.4949, 4.2238)
  line L1170 (15.6639, 4.3214) -> (16.0183, 4.272)
  line L1171 (16.0066, 4.5193) -> (15.6639, 4.3214)
  line L1172 (15.9466, 4.6232) -> (16.0066, 4.5193)
  line L1173 (15.6003, 4.4232) -> (15.9466, 4.6232)
  line L1174 (15.7347, 4.7652) -> (15.6003, 4.4232)
  line L1175 (15.0722, 4.1183) -> (15.4335, 4.3269)
  line L1176 (15.4335, 4.3269) -> (15.623, 4.8091)
  line L1177 (15.623, 4.8091) -> (15.7347, 4.7652)
  arc A27 (13.9257, 16.0823) -> (13.9127, 14.3642) centre (14.8258, 15.2163) ccw
  arc A28 (14.0531, 15.9338) -> (14.0463, 14.5062) centre (14.8258, 15.2163) ccw
  arc A29 (14.2345, 15.8133) -> (14.221, 14.633) centre (14.8258, 15.2163) ccw
  arc A30 (14.3831, 15.6892) -> (14.327, 14.803) centre (14.8258, 15.2163) ccw
  line L1178 (14.0463, 14.5062) -> (14.1218, 14.4228) construction
  line L1179 (14.1218, 14.4228) -> (14.1126, 14.3627) construction
  line L1180 (14.1126, 14.3627) -> (14.0656, 14.3065) construction
  line L1181 (14.0656, 14.3065) -> (14.0039, 14.3026) construction
  line L1182 (14.0039, 14.3026) -> (13.9661, 14.3098) construction
  line L1183 (13.9661, 14.3098) -> (13.9127, 14.3642) construction
  spline S56 degree 4 poles (14.0463, 14.5062) (14.1218, 14.4228) (14.1126, 14.3627) (14.0656, 14.3065) (14.0039, 14.3026) (13.9661, 14.3098) (13.9127, 14.3642) knots 1 1 1 1 1 2 3 4 4 4 4 4
  line L1184 (14.221, 14.633) -> (14.287, 14.5715) construction
  line L1185 (14.287, 14.5715) -> (14.3743, 14.6118) construction
  line L1186 (14.3743, 14.6118) -> (14.4113, 14.6542) construction
  line L1187 (14.4113, 14.6542) -> (14.4121, 14.7281) construction
  line L1188 (14.4121, 14.7281) -> (14.327, 14.803) construction
  spline S57 degree 4 poles (14.221, 14.633) (14.287, 14.5715) (14.3743, 14.6118) (14.4113, 14.6542) (14.4121, 14.7281) (14.327, 14.803) knots 1 1 1 1 1 2 3 3 3 3 3
  line L1189 (14.2345, 15.8133) -> (14.3224, 15.8802) construction
  line L1190 (14.3224, 15.8802) -> (14.4174, 15.7895) construction
  line L1191 (14.4174, 15.7895) -> (14.4151, 15.7335) construction
  line L1192 (14.4151, 15.7335) -> (14.3831, 15.6892) construction
  spline S58 degree 4 poles (14.2345, 15.8133) (14.3224, 15.8802) (14.4174, 15.7895) (14.4151, 15.7335) (14.3831, 15.6892) knots 1 1 1 1 1 2 2 2 2 2
  line L1193 (13.9257, 16.0823) -> (14.0005, 16.1538) construction
  line L1194 (14.0005, 16.1538) -> (14.0891, 16.1176) construction
  line L1195 (14.0891, 16.1176) -> (14.1126, 16.0648) construction
  line L1196 (14.1126, 16.0648) -> (14.1218, 16.0014) construction
  line L1197 (14.1218, 16.0014) -> (14.0531, 15.9338) construction
  spline S59 degree 4 poles (13.9257, 16.0823) (14.0005, 16.1538) (14.0891, 16.1176) (14.1126, 16.0648) (14.1218, 16.0014) (14.0531, 15.9338) knots 1 1 1 1 1 2 3 3 3 3 3
  line L1198 (15.5391, 16.0699) -> (15.5861, 16.1262) construction
  spline S60 degree 4 poles (15.6054, 15.9264) (15.5298, 16.0098) (15.5391, 16.0699) (15.5861, 16.1262) (15.6478, 16.13) (15.6856, 16.1228) (15.739, 16.0685) knots 1 1 1 1 1 2 3 4 4 4 4 4
  line L1199 (15.6054, 15.9264) -> (15.5298, 16.0098) construction
  line L1200 (15.5298, 16.0098) -> (15.5391, 16.0699) construction
  line L1201 (15.5861, 16.1262) -> (15.6478, 16.13) construction
  line L1202 (15.6478, 16.13) -> (15.6856, 16.1228) construction
  line L1203 (15.6856, 16.1228) -> (15.739, 16.0685) construction
  line L1204 (15.4306, 15.7997) -> (15.3646, 15.8611) construction
  spline S61 degree 4 poles (15.4306, 15.7997) (15.3646, 15.8611) (15.2774, 15.8209) (15.2404, 15.7785) (15.2396, 15.7045) (15.3246, 15.6296) knots 1 1 1 1 1 2 3 3 3 3 3
  line L1205 (15.3646, 15.8611) -> (15.2774, 15.8209) construction
  line L1206 (15.2774, 15.8209) -> (15.2404, 15.7785) construction
  line L1207 (15.2404, 15.7785) -> (15.2396, 15.7045) construction
  line L1208 (15.2396, 15.7045) -> (15.3246, 15.6296) construction
  line L1209 (15.4172, 14.6193) -> (15.3292, 14.5524) construction
  spline S62 degree 4 poles (15.4172, 14.6193) (15.3292, 14.5524) (15.2343, 14.6431) (15.2366, 14.6991) (15.2686, 14.7434) knots 1 1 1 1 1 2 2 2 2 2
  line L1210 (15.3292, 14.5524) -> (15.2343, 14.6431) construction
  line L1211 (15.2343, 14.6431) -> (15.2366, 14.6991) construction
  line L1212 (15.2366, 14.6991) -> (15.2686, 14.7434) construction
  arc A31 (15.7259, 14.3504) -> (15.739, 16.0685) centre (14.8258, 15.2163) ccw
  arc A32 (15.5986, 14.4988) -> (15.6054, 15.9264) centre (14.8258, 15.2163) ccw
  arc A33 (15.4172, 14.6193) -> (15.4306, 15.7997) centre (14.8258, 15.2163) ccw
  arc A34 (15.2686, 14.7434) -> (15.3246, 15.6296) centre (14.8258, 15.2163) ccw
  line L1213 (15.7259, 14.3504) -> (15.6512, 14.2789) construction
  spline S63 degree 4 poles (15.7259, 14.3504) (15.6512, 14.2789) (15.5626, 14.3151) (15.5391, 14.3678) (15.5298, 14.4313) (15.5986, 14.4988) knots 1 1 1 1 1 2 3 3 3 3 3
  line L1214 (15.6512, 14.2789) -> (15.5626, 14.3151) construction
  line L1215 (15.5626, 14.3151) -> (15.5391, 14.3678) construction
  line L1216 (15.5391, 14.3678) -> (15.5298, 14.4313) construction
  line L1217 (15.5298, 14.4313) -> (15.5986, 14.4988) construction
  line L1218 (14.7118, -10.7245) -> (14.7118, -11.6041)
  line L1219 (14.8991, -11.6041) -> (14.7118, -11.6041)
  line L1220 (14.8991, -10.7978) -> (14.8991, -11.6041)
  line L1221 (15.8195, -10.7245) -> (15.8195, -11.6041)
  line L1222 (16.0164, -11.6041) -> (16.0164, -10.7345)
  line L1223 (15.8195, -11.6041) -> (16.0164, -11.6041)
  line L1224 (13.5716, -11.6041) -> (13.5716, -9.9507)
  line L1225 (13.7752, -10.2873) -> (13.7752, -10.6919) construction
  spline S64 degree 4 poles (14.7118, -10.7245) (14.7118, -10.2526) (14.3999, -10.0436) (14.0728, -10.0436) (13.7752, -10.2873) (13.7752, -10.6919) knots 1 1 1 1 1 2 3 3 3 3 3
  line L1226 (14.7118, -10.7245) -> (14.7118, -10.2526) construction
  line L1227 (14.7118, -10.2526) -> (14.3999, -10.0436) construction
  line L1228 (14.3999, -10.0436) -> (14.0728, -10.0436) construction
  line L1229 (14.0728, -10.0436) -> (13.7752, -10.2873) construction
  line L1230 (13.7752, -10.6919) -> (13.7752, -11.6041)
  line L1231 (13.7752, -11.6041) -> (13.5716, -11.6041)
  line L1232 (13.5716, -9.9507) -> (13.7752, -9.9507)
  line L1233 (13.7752, -9.9507) -> (13.7752, -10.138)
  line L1234 (14.0728, -9.8243) -> (14.584, -9.8402) construction
  spline S65 degree 3 poles (13.7752, -10.138) (14.0728, -9.8243) (14.584, -9.8402) (14.834, -10.2113) knots 1 1 1 1 2 2 2 2
  line L1235 (13.7752, -10.138) -> (14.0728, -9.8243) construction
  line L1236 (14.584, -9.8402) -> (14.834, -10.2113) construction
  line L1237 (16.0164, -10.1018) -> (16.0164, -10.7345) construction
  spline S66 degree 4 poles (14.834, -10.2113) (15.1227, -9.7823) (15.8128, -9.7823) (16.0164, -10.1018) (16.0164, -10.7345) knots 1 1 1 1 1 2 2 2 2 2
  line L1238 (14.834, -10.2113) -> (15.1227, -9.7823) construction
  line L1239 (15.1227, -9.7823) -> (15.8128, -9.7823) construction
  line L1240 (15.8128, -9.7823) -> (16.0164, -10.1018) construction
  line L1241 (15.8195, -10.7245) -> (15.8195, -10.2738) construction
  spline S67 degree 4 poles (15.8195, -10.7245) (15.8195, -10.2738) (15.5309, -10.0648) (15.2037, -10.0648) (14.8991, -10.2738) (14.8991, -10.7978) knots 1 1 1 1 1 2 3 3 3 3 3
  line L1242 (15.8195, -10.2738) -> (15.5309, -10.0648) construction
  line L1243 (15.5309, -10.0648) -> (15.2037, -10.0648) construction
  line L1244 (15.2037, -10.0648) -> (14.8991, -10.2738) construction
  line L1245 (14.8991, -10.2738) -> (14.8991, -10.7978) construction
  line L1246 (13.5062, -7.2717) -> (13.5062, -8.1513)
  line L1247 (13.6935, -8.1513) -> (13.5062, -8.1513)
  line L1248 (13.6935, -7.345) -> (13.6935, -8.1513)
  line L1249 (14.6139, -7.2717) -> (14.6139, -8.1513)
  line L1250 (14.8107, -8.1513) -> (14.8107, -7.2817)
  line L1251 (14.6139, -8.1513) -> (14.8107, -8.1513)
  line L1252 (12.3659, -8.1513) -> (12.3659, -6.4979)
  line L1253 (12.5695, -6.8345) -> (12.5695, -7.2391) construction
  spline S68 degree 4 poles (13.5062, -7.2717) (13.5062, -6.7998) (13.1943, -6.5908) (12.8671, -6.5908) (12.5695, -6.8345) (12.5695, -7.2391) knots 1 1 1 1 1 2 3 3 3 3 3
  line L1254 (13.5062, -7.2717) -> (13.5062, -6.7998) construction
  line L1255 (13.5062, -6.7998) -> (13.1943, -6.5908) construction
  line L1256 (13.1943, -6.5908) -> (12.8671, -6.5908) construction
  line L1257 (12.8671, -6.5908) -> (12.5695, -6.8345) construction
  line L1258 (12.5695, -7.2391) -> (12.5695, -8.1513)
  line L1259 (12.5695, -8.1513) -> (12.3659, -8.1513)
  line L1260 (12.3659, -6.4979) -> (12.5695, -6.4979)
  line L1261 (12.5695, -6.4979) -> (12.5695, -6.6852)
  line L1262 (12.8671, -6.3715) -> (13.3783, -6.3874) construction
  spline S69 degree 3 poles (12.5695, -6.6852) (12.8671, -6.3715) (13.3783, -6.3874) (13.6283, -6.7585) knots 1 1 1 1 2 2 2 2
  line L1263 (12.5695, -6.6852) -> (12.8671, -6.3715) construction
  line L1264 (13.3783, -6.3874) -> (13.6283, -6.7585) construction
  line L1265 (14.8107, -6.649) -> (14.8107, -7.2817) construction
  spline S70 degree 4 poles (13.6283, -6.7585) (13.9171, -6.3295) (14.6071, -6.3295) (14.8107, -6.649) (14.8107, -7.2817) knots 1 1 1 1 1 2 2 2 2 2
  line L1266 (13.6283, -6.7585) -> (13.9171, -6.3295) construction
  line L1267 (13.9171, -6.3295) -> (14.6071, -6.3295) construction
  line L1268 (14.6071, -6.3295) -> (14.8107, -6.649) construction
  line L1269 (14.6139, -7.2717) -> (14.6139, -6.821) construction
  spline S71 degree 4 poles (14.6139, -7.2717) (14.6139, -6.821) (14.3252, -6.612) (13.9981, -6.612) (13.6935, -6.821) (13.6935, -7.345) knots 1 1 1 1 1 2 3 3 3 3 3
  line L1270 (14.6139, -6.821) -> (14.3252, -6.612) construction
  line L1271 (14.3252, -6.612) -> (13.9981, -6.612) construction
  line L1272 (13.9981, -6.612) -> (13.6935, -6.821) construction
  line L1273 (13.6935, -6.821) -> (13.6935, -7.345) construction
  line L1274 (16.9434, -3.9888) -> (16.9434, -4.8684)
  line L1275 (17.1308, -4.8684) -> (16.9434, -4.8684)
  line L1276 (17.1308, -4.0621) -> (17.1308, -4.8684)
  line L1277 (18.0511, -3.9888) -> (18.0511, -4.8684)
  line L1278 (18.248, -4.8684) -> (18.248, -3.9989)
  line L1279 (18.0511, -4.8684) -> (18.248, -4.8684)
  line L1280 (15.8032, -4.8684) -> (15.8032, -3.2151)
  line L1281 (16.0068, -3.5517) -> (16.0068, -3.9562) construction
  spline S72 degree 4 poles (16.9434, -3.9888) (16.9434, -3.517) (16.6316, -3.308) (16.3044, -3.308) (16.0068, -3.5517) (16.0068, -3.9562) knots 1 1 1 1 1 2 3 3 3 3 3
  line L1282 (16.9434, -3.9888) -> (16.9434, -3.517) construction
  line L1283 (16.9434, -3.517) -> (16.6316, -3.308) construction
  line L1284 (16.6316, -3.308) -> (16.3044, -3.308) construction
  line L1285 (16.3044, -3.308) -> (16.0068, -3.5517) construction
  line L1286 (16.0068, -3.9562) -> (16.0068, -4.8684)
  line L1287 (16.0068, -4.8684) -> (15.8032, -4.8684)
  line L1288 (15.8032, -3.2151) -> (16.0068, -3.2151)
  line L1289 (16.0068, -3.2151) -> (16.0068, -3.4024)
  line L1290 (16.3044, -3.0887) -> (16.8156, -3.1045) construction
  spline S73 degree 3 poles (16.0068, -3.4024) (16.3044, -3.0887) (16.8156, -3.1045) (17.0656, -3.4757) knots 1 1 1 1 2 2 2 2
  line L1291 (16.0068, -3.4024) -> (16.3044, -3.0887) construction
  line L1292 (16.8156, -3.1045) -> (17.0656, -3.4757) construction
  line L1293 (18.248, -3.3661) -> (18.248, -3.9989) construction
  spline S74 degree 4 poles (17.0656, -3.4757) (17.3544, -3.0466) (18.0444, -3.0466) (18.248, -3.3661) (18.248, -3.9989) knots 1 1 1 1 1 2 2 2 2 2
  line L1294 (17.0656, -3.4757) -> (17.3544, -3.0466) construction
  line L1295 (17.3544, -3.0466) -> (18.0444, -3.0466) construction
  line L1296 (18.0444, -3.0466) -> (18.248, -3.3661) construction
  line L1297 (18.0511, -3.9888) -> (18.0511, -3.5382) construction
  spline S75 degree 4 poles (18.0511, -3.9888) (18.0511, -3.5382) (17.7625, -3.3291) (17.4353, -3.3291) (17.1308, -3.5381) (17.1308, -4.0621) knots 1 1 1 1 1 2 3 3 3 3 3
  line L1298 (18.0511, -3.5382) -> (17.7625, -3.3291) construction
  line L1299 (17.7625, -3.3291) -> (17.4353, -3.3291) construction
  line L1300 (17.4353, -3.3291) -> (17.1308, -3.5381) construction
  line L1301 (17.1308, -3.5381) -> (17.1308, -4.0621) construction
  arc A35 (15.0722, 4.1183) -> (14.894, 4.2212) centre (14.834, 3.9115) ccw
  arc A36 (15.1322, 3.8086) -> (15.1322, 4.0144) centre (14.834, 3.9115) ccw
  arc A37 (14.894, 3.6018) -> (15.0722, 3.7047) centre (14.834, 3.9115) ccw
  arc A38 (14.5958, 3.7047) -> (14.774, 3.6018) centre (14.834, 3.9115) ccw
  arc A39 (14.774, 4.2212) -> (14.5958, 4.1183) centre (14.834, 3.9115) ccw
  arc A40 (14.5358, 4.0144) -> (14.5358, 3.8086) centre (14.834, 3.9115) ccw
  point P0 (0, 0)
  point P1 (-19.2759, 1.9324)
  point P2 (-12.5396, 11.56)
  point P3 (-5.2257, 11.56)
  point P4 (2.0231, 11.56)
  point P5 (14.0765, 8.8227)
  point P6 (14.0114, 9.8408)
  point P7 (-0.3803, 16.0471)
  point P8 (-11.5059, 16.0552)
  point P9 (-12.467, 0.2627)
  point P10 (0.084, 15.8353)
  point P11 (-6.5621, 13.8643)
  point P12 (-5.6499, -1.9282)
  point P13 (10.0775, -1.9038)
  point P14 (3.0486, -0.2423)
  point P15 (15.8032, -3.2151)
  point P16 (17.1634, -11.6122)
  point P17 (17.1634, -9.4213)
  point P18 (13.7915, -4.8684)
  point P19 (12.3661, -6.4974)
  point P20 (13.5716, -9.9507)
  point P21 (-3.9151, -0.2667)
  point P22 (16.072, -7.6376)
  point P23 (10.1798, 13.4974)
  point P24 (-14.6823, -4.054)
  point P25 (-9.486, -4.054)
  point P26 (-4.2979, -4.054)
  point P27 (1.8025, -4.054)
  point P28 (6.9907, -4.054)
  point P29 (11.5517, 15.5081)
  point P30 (18.7199, 16.038)
  point P31 (19.3461, 15.9168)
  point P32 (19.8185, 15.9168)
  point P33 (19.8185, 15.4688)
  point P34 (19.3461, 15.4688)
  point P35 (19.4602, 14.5077)
  point P36 (19.7045, 14.5077)
  point P37 (19.3624, 14.3856)
  point P38 (19.7941, 14.0191)
  point P39 (15.114, 5.1174)
  point P40 (14.545, 5.1184)
  point P41 (13.9297, 4.757)
  point P42 (13.6443, 4.2647)
  point P43 (13.6496, 3.5511)
  point P44 (13.9333, 3.0578)
  point P45 (14.554, 2.7056)
  point P46 (15.1229, 2.7046)
  point P47 (15.7383, 3.0661)
  point P48 (16.0236, 3.5583)
  point P49 (16.0183, 4.272)
  point P50 (15.7347, 4.7652)
  point P51 (13.5716, -9.9507)
  point P52 (12.3659, -6.4979)
  point P53 (15.7026, -8.9332)
  point P54 (15.8032, -3.2151)
  point P55 (19.1399, -5.6503)
  dimension "d11" = 360
  dimension "d12" = 360
  constraints: 1764 end point, 64 point on circle, 57 coincident, 41 centre point, 10 point on line, 590 other
extrude "Extrusion3" add sketch "Sketch3" along normal blind 0.01 separate body
sketch "Sketch5" plane through (0, 0, 1.2) normal (0, 0, 1) x (1, 0, 0)
  line L0 (-21.39, 20.9) -> (-20.14, 20.9)
  line L1 (-20.14, 20.9) -> (-20.14, 18.5)
  line L2 (-20.14, 18.5) -> (-21.39, 18.5)
  line L3 (-21.39, 18.5) -> (-21.39, 20.9)
  line L4 (-18.85, 20.9) -> (-17.6, 20.9)
  line L5 (-17.6, 20.9) -> (-17.6, 18.5)
  line L6 (-17.6, 18.5) -> (-18.85, 18.5)
  line L7 (-18.85, 18.5) -> (-18.85, 20.9)
  line L8 (17.6, 20.9) -> (18.85, 20.9)
  line L9 (18.85, 20.9) -> (18.85, 18.5)
  line L10 (18.85, 18.5) -> (17.6, 18.5)
  line L11 (17.6, 18.5) -> (17.6, 20.9)
  line L12 (20.14, 20.9) -> (21.39, 20.9)
  line L13 (21.39, 20.9) -> (21.39, 18.5)
  line L14 (21.39, 18.5) -> (20.14, 18.5)
  line L15 (20.14, 18.5) -> (20.14, 20.9)
  line L16 (-5.715, -18.5) -> (-4.445, -18.5)
  line L17 (-4.445, -18.5) -> (-4.445, -20.9)
  line L18 (-4.445, -20.9) -> (-5.715, -20.9)
  line L19 (-5.715, -20.9) -> (-5.715, -18.5)
  line L20 (-3.175, -18.5) -> (-1.905, -18.5)
  line L21 (-1.905, -18.5) -> (-1.905, -20.9)
  line L22 (-1.905, -20.9) -> (-3.175, -20.9)
  line L23 (-3.175, -20.9) -> (-3.175, -18.5)
  line L24 (-0.635, -18.5) -> (0.635, -18.5)
  line L25 (0.635, -18.5) -> (0.635, -20.9)
  line L26 (0.635, -20.9) -> (-0.635, -20.9)
  line L27 (-0.635, -20.9) -> (-0.635, -18.5)
  line L28 (1.905, -18.5) -> (3.175, -18.5)
  line L29 (3.175, -18.5) -> (3.175, -20.9)
  line L30 (3.175, -20.9) -> (1.905, -20.9)
  line L31 (1.905, -20.9) -> (1.905, -18.5)
  line L32 (4.445, -18.5) -> (5.715, -18.5)
  line L33 (5.715, -18.5) -> (5.715, -20.9)
  line L34 (5.715, -20.9) -> (4.445, -20.9)
  line L35 (4.445, -20.9) -> (4.445, -18.5)
  line L36 (23.765, 20.5) -> (-23.765, 20.5) projected
  line L37 (-23.765, -20.5) -> (23.765, -20.5) projected
  point P0 (0, 0)
  dimension "d35" = 0.4
  dimension "d36" = 0.4
  constraints: 72 end point, 14 collinear, 2 horizontal
  measures "d35" distance between parallel lines of L36 L0
  measures "d36" distance between parallel lines of L37 L18
extrude "Extrusion4" add sketch "Sketch5" along normal blind 0.3 separate body